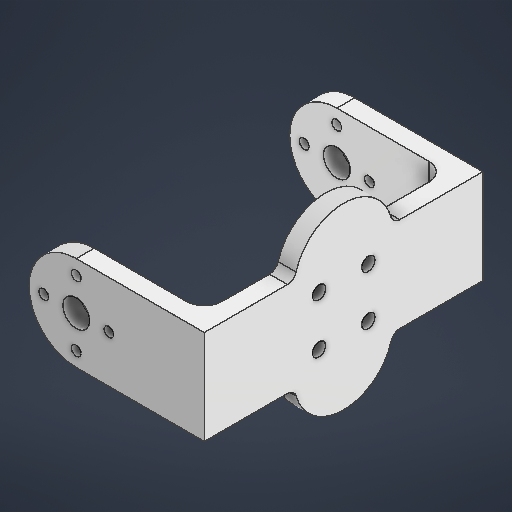
# Autodesk Inventor part: L2
Saved by Autodesk Inventor 2026.1 (Build 301233000, 233)
## iProperties
Created: 2025-09-17
Part Number: L2
Material: Generic
Document SubType Name: Modeling
Designer: emanuel
Density: 1 g/cm^3
Appearance: Default
Author: emanuel
Autodesk Inventor part; units mm, degrees
ref_plane "YZ Plane" through (0, 0, 0) normal (1, 0, 0) x (0, 1, 0)
ref_plane "XZ Plane" through (0, 0, 0) normal (0, 1, 0) x (-1, 0, 0)
ref_plane "XY Plane" through (0, 0, 0) normal (0, 0, 1) x (1, 0, 0)
sketch "Sketch1" plane through (0, 0, 0) normal (0, 1, 0) x (-1, 0, 0)
  line L0 (0, 0) -> (0, -58)
  line L1 (0, -58) -> (35, -58)
  line L2 (35, -58) -> (35, -62)
  line L3 (35, -62) -> (-4, -62)
  line L4 (-4, -62) -> (-4, 0)
  line L5 (-4, 0) -> (0, 0)
  line L6 (0, 0) -> (35, 0)
  line L7 (35, 0) -> (35, -4)
  line L8 (35, -4) -> (0, -4)
  line L9 (0, -4) -> (0, 0)
  dimension "d0" = 58
  dimension "d1" = 35
  dimension "d2" = 4
  dimension "d3" = 39
  dimension "d27" = 35
  dimension "d28" = 4
  constraints: 20 end point, 5 perpendicular, 3 parallel, 1 horizontal, 1 vertical
  measures "d0" distance of L0.start L0.end
  measures "d1" distance of L0.end L1.end
  measures "d2" distance of L1.end L2.end
  measures "d3" distance of L2.end L3.end
  measures "d27" distance of L7.end L8.end
  measures "d28" distance of L6.end L7.end
extrude "Extrusion1" add sketch "Sketch1" along normal blind 21
sketch "Sketch2" plane through (4, 0, 0) normal (1, 0, 0) x (0, 0, -1)
  line L0 (0, 21) -> (62, 21) projected
  line L1 (0, 21) -> (25.5, 21)
  line L2 (25.5, 21) -> (25.5, 16)
  line L3 (25.5, 16) -> (0, 16)
  line L4 (0, 16) -> (0, 21)
  line L5 (25.5, 16) -> (36.5, 16)
  line L6 (36.5, 16) -> (36.5, 5)
  line L7 (36.5, 5) -> (25.5, 5)
  line L8 (25.5, 5) -> (25.5, 16)
  circle A0 centre (25.5, 16) radius 1.5
  circle A1 centre (36.5, 16) radius 1.5
  circle A2 centre (25.5, 5) radius 1.5
  circle A3 centre (36.5, 5) radius 1.5
  point P0 (0, 0)
  dimension "d6" = 25.5
  dimension "d7" = 5
  dimension "d8" = 11
  dimension "d9" = 11
  dimension "d10" = 3
  dimension "d11" = 3
  dimension "d12" = 3
  dimension "d13" = 3
  constraints: 16 end point, 4 centre point, 4 coincident, 4 parallel, 2 horizontal, 2 perpendicular
  measures "d6" distance of L2.end L3.end
  measures "d7" distance of L1.end L2.end
  measures "d8" distance of L6.end L7.end
  measures "d9" distance of L5.end L6.end
  measures "d10" diameter of A0
  measures "d11" diameter of A1
  measures "d12" diameter of A2
  measures "d13" diameter of A3
extrude "Extrusion2" cut sketch "Sketch2" against normal blind 21 contours A0 L5 L2 | L2 L3 A0 | L3 L8 A0 | L5 A0 L8 | A1 L6 L5 | L5 L6 A1 | A2 L7 L8 | L8 L7 A2 | A3 L7 L6 | L6 L7 A3
sketch "Sketch3" plane through (-35, 0, -58) normal (0, 0, 1) x (1, 0, 0)
  line L0 (0, 0) -> (0, 21) projected
  line L1 (0, 10.5) -> (10.5, 10.5)
  circle A0 centre (10.5, 10.5) radius 10.5
  line L2 (0, 21) -> (10.5, 21)
  line L3 (10.5, 21) -> (10.5, 0)
  line L4 (10.5, 0) -> (0, 0)
  line L5 (0, 0) -> (0, 21)
  circle A1 centre (10.5, 10.5) radius 8
  circle A2 centre (10.5, 10.5) radius 6.5
  line L6 (10.5, 18.5) -> (10.5, 17)
  line L7 (10.5, 4) -> (10.5, 2.5)
  line L8 (2.5, 10.5) -> (4, 10.5)
  line L9 (10.5, 10.5) -> (18.5, 10.5)
  line L10 (18.5, 10.5) -> (17, 10.5)
  circle A3 centre (10.5, 17.75) radius 1.1
  circle A4 centre (3.25, 10.5) radius 1.1
  circle A5 centre (17.75, 10.5) radius 1.1
  circle A6 centre (10.5, 3.25) radius 1.1
  circle A7 centre (10.5, 10.5) radius 3
  point P0 (35, 0)
  point P1 (10.5, 21)
  dimension "d16" = 10.5
  dimension "d17" = 16
  dimension "d18" = 13
  dimension "d19" = 2.2
  dimension "d20" = 2.2
  dimension "d21" = 2.2
  dimension "d22" = 2.2
  dimension "d23" = 6
  constraints: 20 end point, 10 point on circle, 8 centre point, 8 point on line, 5 midpoint, 4 coincident, 2 horizontal, 2 parallel, 1 perpendicular
  measures "d16" distance of L1.start L1.end
  measures "d17" diameter of A1
  measures "d18" diameter of A2
  measures "d19" diameter of A3
  measures "d20" diameter of A4
  measures "d21" diameter of A5
  measures "d22" diameter of A6
  measures "d23" diameter of A7
extrude "Extrusion3" cut sketch "Sketch3" along normal mid plane 1000 contours L0 A0 L4 | L0 L2 A0 | A4 A1 L1 | L1 A1 A4 | A6 A1 L3 | L3 A1 A6 | A1 A4 A2 L1 | L1 A2 A4 A1 | A3 A1 L3 | L3 A1 A3 | A1 A6 A2 L3 | L3 A2 A6 A1 | A2 A4 L1 | L1 A4 A2 | A1 L3 A2 A3 | A1 A3 A2 L3 | A2 A6 L3 | L3 A6 A2 | A5 A2 L9 A1 | A1 A5 | A2 L3 A3 | A2 A3 L3 | A1 L9 A2 A5 | A5 L9 A2 | A7 L3 L1 | L1 L3 A7 | A2 L9 A5 | L3 L9 A7 | L3 A7 L9
fillet "Fillet1" radius 4 2 edges at (0, 10.5, -58) (0, 10.5, -4)
sketch "Sketch4" plane through (4, 0, 0) normal (1, 0, 0) x (0, 0, -1)
  circle A0 centre (25.5, 16) radius 1.5 projected
  line L0 (25.5, 16) -> (20.5, 16)
  line L1 (20.5, 16) -> (41.5, 16)
  line L2 (20.5, 16) -> (41.5, 16)
  line L3 (41.5, 16) -> (41.5, 31)
  line L4 (41.5, 31) -> (20.5, 31)
  line L5 (20.5, 31) -> (20.5, 16)
  circle A1 centre (25.5, 5) radius 1.5 projected
  line L6 (25.5, 5) -> (20.5, 5)
  circle A2 centre (36.5, 5) radius 1.5 projected
  line L7 (20.5, 5) -> (36.5, 5)
  line L8 (36.5, 5) -> (41.5, 5)
  line L9 (20.5, 5) -> (41.5, 5)
  line L10 (41.5, 5) -> (41.5, -10)
  line L11 (41.5, -10) -> (20.5, -10)
  line L12 (20.5, -10) -> (20.5, 5)
  line L13 (0, 21) -> (62, 21) projected
  line L14 (20.5, 31) -> (41.5, 31)
  line L15 (41.5, 31) -> (41.5, 21)
  line L16 (41.5, 21) -> (20.5, 21)
  line L17 (20.5, 21) -> (20.5, 31)
  line L18 (41.5, -10) -> (20.5, -10)
  line L19 (20.5, -10) -> (20.5, -2.5)
  line L20 (41.5, -2.5) -> (41.5, -10)
  line L21 (20.5, -10) -> (41.5, -10)
  line L22 (41.5, -10) -> (41.5, 0)
  line L23 (41.5, 0) -> (20.5, 0)
  line L24 (20.5, 0) -> (20.5, -10)
  line L25 (20.5, 31) -> (41.5, 31)
  line L26 (41.5, 31) -> (41.5, 21)
  line L27 (41.5, 21) -> (20.5, 21)
  line L28 (20.5, 21) -> (20.5, 31)
  point P0 (0, 0)
  point P1 (38, 5)
  point P2 (35, 5)
  point P3 (27, 5)
  point P4 (24, 5)
  dimension "d29" = 5
  dimension "d30" = 21
  dimension "d31" = 15
  dimension "d32" = 15
  constraints: 56 end point, 11 parallel, 8 horizontal, 6 perpendicular, 5 point on line, 1 collinear, 1 midpoint
  measures "d29" distance of L0.start L0.end
  measures "d30" distance of L0.end L1.end
  measures "d31" distance of L3.end L2.end
  measures "d32" distance of L9.end L10.end
extrude "Extrusion4" add sketch "Sketch4" against normal blind 4 contours L13 L5 L4 L3 | L7 A2 L8 L10 L23 L12 L6 A1 | L23 L10 L11 L12
fillet "Fillet2" radius 2 4 edges at (2, 21, -41.5) (2, 21, -20.5) (2, 0, -41.5) (2, 0, -20.5)
fillet "Fillet3" radius 11 4 edges at (2, 31, -20.5) (2, 31, -41.5) (2, -10, -20.5) (2, -10, -41.5)
body "Solid1"
